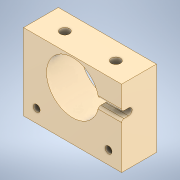
# Autodesk Inventor part: Soporte Motor Izq
Saved by Autodesk Inventor 2021 (Build 250183000, 183)
## iProperties
Created: 2023-01-27
Part Number: Soporte Motor Izq
Material: Polietileno, baja densidad
Document SubType Name: Modeling
Designer: Diego.labarca
Density: 0.894 g/cm^3
Appearance: Suave - Color hueso
Author: Diego.labarca
Autodesk Inventor part; units mm, degrees
ref_plane "YZ Plane" through (0, 0, 0) normal (1, 0, 0) x (0, 1, 0)
ref_plane "XZ Plane" through (0, 0, 0) normal (0, 1, 0) x (-1, 0, 0)
ref_plane "XY Plane" through (0, 0, 0) normal (0, 0, 1) x (1, 0, 0)
sketch "Boceto16" plane through (0, 0, 0) normal (0, 0, 1) x (1, 0, 0)
  line L0 (-21.15, 21.15) -> (21.15, 21.15)
  line L1 (21.15, 21.15) -> (21.15, -21.15)
  line L2 (21.15, -21.15) -> (-21.15, -21.15)
  line L3 (-21.15, -21.15) -> (-21.15, 21.15)
  line L4 (2.3235, 0) -> (0, 0)
  line L5 (0, 0) -> (0, 2.4447)
  dimension "d75" = 42.3
  dimension "d76" = 42.3
  constraints: 12 end point, 2 horizontal, 2 parallel, 2 perpendicular, 2 other
  measures "d75" distance of L1.end L2.end
  measures "d76" distance of L0.end L1.end
extrude "Extrusión15" add sketch "Boceto16" along normal blind 15
sketch "Boceto17" plane through (0, 0, 15) normal (0, 0, 1) x (1, 0, 0)
  circle A0 centre (15.5, 15.5) radius 1.5
  point P0 (0, 0)
  dimension "d79" = 3
  dimension "d80" = 15.5
  dimension "d81" = 15.5
  constraints: 1 centre point
  measures "d79" diameter of A0
  measures "d80" horizontal distance of point (0, 0) A0.centre
  measures "d81" horizontal distance of point (0, 0) A0.centre
extrude "Extrusión16" cut sketch "Boceto17" against normal through all
pattern_linear "Patrón rectangular2" count 2 spacing 31 along (-1, 0, 0) count 2 spacing 31 along (0, -1, 0) of "Extrusión16"
sketch "Boceto18" plane through (0, 0, 15) normal (0, 0, 1) x (1, 0, 0)
  line L0 (-21.15, -21.15) -> (21.15, -21.15) projected
  line L1 (-21.15, 21.15) -> (-21.15, -21.15) projected
  line L2 (21.15, -21.15) -> (-21.15, -21.15)
  line L3 (-21.15, -21.15) -> (-21.15, 11.85)
  line L4 (-21.15, 11.85) -> (21.15, 11.85)
  line L5 (21.15, 11.85) -> (21.15, -21.15)
  circle A0 centre (-15.5, -15.5) radius 1.5 projected
  circle A1 centre (15.5, -15.5) radius 1.5 projected
  circle A2 centre (-15.5, 15.5) radius 1.5 projected
  circle A3 centre (15.5, 15.5) radius 1.5 projected
  line L6 (-21.15, -21.15) -> (21.15, -21.15) projected
  line L7 (21.15, -21.15) -> (21.15, 21.15) projected
  line L8 (21.15, 21.15) -> (-21.15, 21.15) projected
  line L9 (-21.15, 21.15) -> (-21.15, -21.15) projected
  point P0 (0, 0)
  point P1 (21.15, 11.85)
  dimension "d90" = 33
  constraints: 8 end point, 2 parallel, 1 horizontal, 1 perpendicular, 1 point on line
  measures "d90" distance of L2.end L3.end
extrude "Extrusión17" cut sketch "Boceto18" against normal through all contours L1 L8 L7 L4
sketch "Boceto19" plane through (0, 0, 15) normal (0, 0, 1) x (1, 0, 0)
  circle A0 centre (0, 0) radius 11.25
  dimension "d93" = 22.5
  constraints: 1 centre point, 1 coincident
  measures "d93" diameter of A0
extrude "Extrusión18" cut sketch "Boceto19" against normal through all
sketch "Boceto20" plane through (21.15, -21.15, 15) normal (1, 0, 0) x (0, 0, -1)
  line L0 (0, 0) -> (0, 33) projected
  circle A0 centre (0, 21.15) radius 1.5
  circle A1 centre (3, 21.15) radius 1.5
  line L1 (15, 33) -> (0, 33) projected
  line L2 (3, 22.65) -> (0, 22.65)
  line L3 (0, 19.65) -> (3, 19.65)
  line L4 (0, 9.9) -> (0, 32.4) projected
  line L5 (3, 21.15) -> (2.4132, 21.15)
  line L6 (15, 21.15) -> (14.0554, 21.15)
  dimension "d99" = 3
  dimension "d102" = 3
  dimension "d103" = 3
  constraints: 8 end point, 4 point on circle, 3 point on line, 2 centre point, 2 horizontal, 2 tangent, 1 collinear
  measures "d99" diameter of A0
  measures "d102" diameter of A1
  measures "d103" distance of L3.start L3.end
extrude "Extrusión19" cut sketch "Boceto20" against normal up to surface contours L0 A0 | A0 A1 L3 | L2 A1 A0 | A1 picked at (0.2169, 21.6005)
fillet "Empalme3" radius 1 2 edges at (16.1498, 1.5, 15) (16.1498, -1.5, 15)
sketch "Boceto21" plane through (-21.15, 11.85, 15) normal (0, 1, 0) x (1, 0, 0)
  circle A0 centre (32.3, 7.5) radius 2
  circle A1 centre (10.3, 7.5) radius 2
  line L0 (0, 15) -> (42.3, 15) projected
  line L1 (42.3, 15) -> (42.3, 0) projected
  line L2 (0, 0) -> (0, 15) projected
  point P0 (21.15, 15)
  dimension "d105" = 4
  dimension "d106" = 4
  dimension "d107" = 7.5
  dimension "d108" = 7.5
  dimension "d111" = 10
  dimension "d115" = 32
  constraints: 2 centre point
  measures "d105" diameter of A0
  measures "d106" diameter of A1
  measures "d107" distance from line of L0 A1.centre
  measures "d108" distance from line of A0.centre L0
  measures "d111" distance from line of A0.centre L1
  measures "d115" distance from line of L1 A1.centre
extrude "Extrusión20" cut sketch "Boceto21" against normal blind 5
equation "\"d102\" = d99"
equation "\"d106\" = d105"
equation "\"d107\" = d108"
